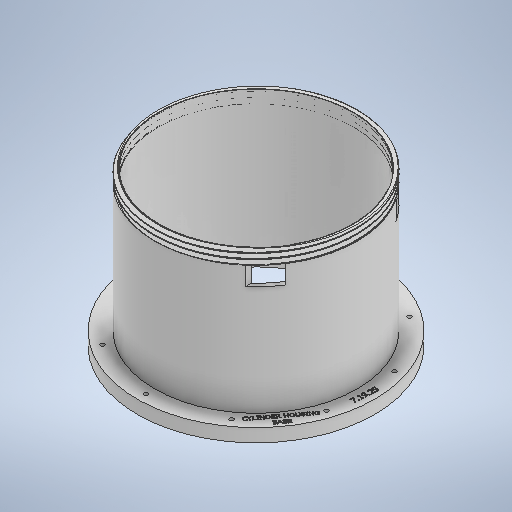
# Autodesk Inventor part: Cylinder Housing_base
Saved by Autodesk Inventor 2025 (Build 290162000, 162)
## iProperties
Created: 2025-07-09
Part Number: Cylinder Housing_base
Material: Generic
Document SubType Name: Modeling
Designer: mumin
Density: 1 g/cm^3
Appearance: Default
Author: mumin
Autodesk Inventor part; units mm, degrees
ref_plane "YZ Plane" through (0, 0, 0) normal (1, 0, 0) x (0, 1, 0)
ref_plane "XZ Plane" through (0, 0, 0) normal (0, 1, 0) x (-1, 0, 0)
ref_plane "XY Plane" through (0, 0, 0) normal (0, 0, 1) x (1, 0, 0)
sketch "Sketch1" plane through (0, 0, 0) normal (0, 0, 1) x (1, 0, 0)
  line L0 (110, 0) -> (110, 175)
  line L1 (110, 0) -> (135, 0)
  line L2 (135, 0) -> (135, 15)
  line L3 (135, 15) -> (115, 15)
  line L4 (115, 15) -> (115, 175)
  line L5 (0, -40) -> (0, 240) projected
  line L6 (-27, 0) -> (162, 0) projected
  line L7 (0, 200) -> (0, 195)
  line L8 (110, 175) -> (115, 175)
  point P0 (0, 0)
  point P1 (115, 132.5)
  point P2 (110, 157.9951)
  point P3 (110, 127.5)
  point P4 (112.5, 175)
  dimension "d0" = 135
  dimension "d1" = 110
  dimension "d2" = 115
  dimension "d3" = 15
  dimension "d24" = 175
  constraints: 14 end point, 6 point on line, 4 perpendicular, 1 collinear, 1 horizontal, 1 midpoint, 1 vertical
  measures "d0" distance between parallel lines of L5 L2
  measures "d1" distance between parallel lines of L5 L0
  measures "d2" distance between parallel lines of L5 L4
  measures "d3" distance of L1.end L2.end
  measures "d24" distance from line of L6 point (112.5, 175)
revolve "Revolution1" add sketch "Sketch1" angle 360 about axis through (0, -10, 0) along (0, 1, 0)
sketch "Sketch3" plane through (0, 15, 0) normal (0, 1, 0) x (1, 0, 0)
  point P0 (0, 0)
  point P1 (0, -125)
  dimension "d11" = 125
  measures "d11" distance of point (0, 0) point (0, -125)
hole "Hole1" at (0, 15, 125) direction (0, -1, 0) diameter 4.5 depth 15
pattern_circular "Circular Pattern1" count 10 over 360 about axis through (0, -10, 0) along (0, 1, 0) of "Hole1"
sketch "Sketch4" plane through (0, 15, 0) normal (0, 1, 0) x (1, 0, 0)
  line L0 (76.2861, -94.0142) -> (115.6188, -42.2704) construction
  line L1 (115.6188, -42.2704) -> (120.4379, -45.9335) construction
  line L2 (120.4379, -45.9335) -> (81.1052, -97.6773) construction
  line L3 (81.1052, -97.6773) -> (76.2861, -94.0142) construction
  line L4 (120.7443, -14.9348) -> (122.6586, 12.509) construction
  line L5 (122.6586, 12.509) -> (135.1331, 11.6389) construction
  line L6 (135.1331, 11.6389) -> (133.2188, -15.805) construction
  line L7 (133.2188, -15.805) -> (120.7443, -14.9348) construction
  spline S0 degree 2 poles (82.4542, -94.4835) (82.16, -94.8706) (81.401, -95.3268) (80.9582, -95.3669) knots 0 0 0 1 2 2 2
  spline S1 degree 2 poles (80.9582, -95.3669) (80.5187, -95.4094) (79.5459, -95.0822) (79.0427, -94.6997) knots 0 0 0 1 2 2 2
  spline S2 degree 2 poles (79.0427, -94.6997) (78.5427, -94.3196) (77.9945, -93.5009) (77.9042, -93.0505) knots 0 0 0 1 2 2 2
  spline S3 degree 2 poles (77.9042, -93.0505) (77.818, -92.6083) (78.0326, -91.7434) (78.3391, -91.3402) knots 0 0 0 1 2 2 2
  spline S4 degree 2 poles (78.3391, -91.3402) (78.4911, -91.1402) (78.8165, -90.8327) (78.9744, -90.7186) knots 0 0 0 1 2 2 2
  spline S5 degree 2 poles (78.9744, -90.7186) (79.1144, -90.6215) (79.4373, -90.4445) (79.6088, -90.3662) knots 0 0 0 1 2 2 2
  line L8 (79.6088, -90.3662) -> (80.2475, -90.8517)
  line L9 (80.2475, -90.8517) -> (80.2156, -90.8936)
  spline S6 degree 2 poles (80.2156, -90.8936) (80.0972, -90.9155) (79.7498, -90.9976) (79.5425, -91.0894) knots 0 0 0 1 2 2 2
  spline S7 degree 2 poles (79.5425, -91.0894) (79.3434, -91.1773) (78.9648, -91.4544) (78.7883, -91.6867) knots 0 0 0 1 2 2 2
  spline S8 degree 2 poles (78.7883, -91.6867) (78.5946, -91.9415) (78.4585, -92.5557) (78.5285, -92.8787) knots 0 0 0 1 2 2 2
  spline S9 degree 2 poles (78.5285, -92.8787) (78.6043, -93.2009) (79.0782, -93.8563) (79.462, -94.1481) knots 0 0 0 1 2 2 2
  spline S10 degree 2 poles (79.462, -94.1481) (79.8717, -94.4595) (80.6116, -94.7115) (80.9447, -94.695) knots 0 0 0 1 2 2 2
  spline S11 degree 2 poles (80.9447, -94.695) (81.269, -94.6768) (81.8098, -94.3805) (82.0011, -94.1289) knots 0 0 0 1 2 2 2
  spline S12 degree 2 poles (82.0011, -94.1289) (82.1752, -93.8998) (82.359, -93.4237) (82.3903, -93.2083) knots 0 0 0 1 2 2 2
  spline S13 degree 2 poles (82.3903, -93.2083) (82.4168, -92.9994) (82.4069, -92.6509) (82.3922, -92.543) knots 0 0 0 1 2 2 2
  line L10 (82.3922, -92.543) -> (82.4216, -92.5043)
  line L11 (82.4216, -92.5043) -> (83.0539, -92.9849)
  spline S14 degree 2 poles (83.0539, -92.9849) (83.0146, -93.1637) (82.951, -93.4818) (82.8775, -93.6856) knots 0 0 0 1 2 2 2
  spline S15 degree 2 poles (82.8775, -93.6856) (82.8032, -93.9039) (82.6357, -94.2448) (82.4542, -94.4835) knots 0 0 0 1 2 2 2
  line L12 (81.838, -86.8845) -> (83.0348, -89.9166)
  line L13 (83.0348, -89.9166) -> (84.796, -91.2554)
  line L14 (84.796, -91.2554) -> (84.3939, -91.7845)
  line L15 (84.3939, -91.7845) -> (82.6875, -90.4873)
  line L16 (82.6875, -90.4873) -> (79.3909, -90.1038)
  line L17 (79.3909, -90.1038) -> (79.8372, -89.5167)
  line L18 (79.8372, -89.5167) -> (82.3709, -89.8192)
  line L19 (82.3709, -89.8192) -> (81.4113, -87.4458)
  line L20 (81.4113, -87.4458) -> (81.838, -86.8845)
  line L21 (87.8512, -87.2362) -> (86.0981, -89.5426)
  line L22 (86.0981, -89.5426) -> (82.1175, -86.5168)
  line L23 (82.1175, -86.5168) -> (82.5196, -85.9878)
  line L24 (82.5196, -85.9878) -> (86.0292, -88.6556)
  line L25 (86.0292, -88.6556) -> (87.3803, -86.8782)
  line L26 (87.3803, -86.8782) -> (87.8512, -87.2362)
  line L27 (89.2219, -85.433) -> (88.0499, -86.9749)
  line L28 (88.0499, -86.9749) -> (87.6434, -86.666)
  line L29 (87.6434, -86.666) -> (88.0284, -86.1595)
  line L30 (88.0284, -86.1595) -> (84.8607, -83.7516)
  line L31 (84.8607, -83.7516) -> (84.4758, -84.2581)
  line L32 (84.4758, -84.2581) -> (84.0693, -83.9491)
  line L33 (84.0693, -83.9491) -> (85.2414, -82.4072)
  line L34 (85.2414, -82.4072) -> (85.6478, -82.7162)
  line L35 (85.6478, -82.7162) -> (85.2629, -83.2226)
  line L36 (85.2629, -83.2226) -> (88.4305, -85.6305)
  line L37 (88.4305, -85.6305) -> (88.8155, -85.1241)
  line L38 (88.8155, -85.1241) -> (89.2219, -85.433)
  line L39 (91.8848, -81.9299) -> (91.4336, -82.5234)
  line L40 (91.4336, -82.5234) -> (86.6627, -81.6757)
  line L41 (86.6627, -81.6757) -> (90.0948, -84.2847)
  line L42 (90.0948, -84.2847) -> (89.7197, -84.7782)
  line L43 (89.7197, -84.7782) -> (85.7391, -81.7524)
  line L44 (85.7391, -81.7524) -> (86.3104, -81.0008)
  line L45 (86.3104, -81.0008) -> (90.6806, -81.7933)
  line L46 (90.6806, -81.7933) -> (87.5291, -79.3976)
  line L47 (87.5291, -79.3976) -> (87.9043, -78.9041)
  line L48 (87.9043, -78.9041) -> (91.8848, -81.9299)
  spline S16 degree 2 poles (92.8966, -76.4744) (93.4417, -76.8888) (93.9832, -77.9977) (93.9463, -78.555) knots 0 0 0 1 2 2 2
  spline S17 degree 2 poles (93.9463, -78.555) (93.9062, -79.0028) (93.562, -79.7235) (93.1942, -80.2073) knots 0 0 0 1 2 2 2
  line L49 (93.1942, -80.2073) -> (92.4978, -81.1235)
  line L50 (92.4978, -81.1235) -> (88.5173, -78.0977)
  line L51 (88.5173, -78.0977) -> (89.2063, -77.1913)
  spline S18 degree 2 poles (89.2063, -77.1913) (89.6329, -76.63) (90.2862, -76.1188) (90.6062, -76.0058) knots 0 0 0 1 2 2 2
  spline S19 degree 2 poles (90.6062, -76.0058) (91.1528, -75.8156) (92.3159, -76.033) (92.8966, -76.4744) knots 0 0 0 1 2 2 2
  spline S20 degree 2 poles (92.4708, -77.0211) (92.0128, -76.6729) (91.1339, -76.4833) (90.722, -76.6435) knots 0 0 0 1 2 2 2
  spline S21 degree 2 poles (90.722, -76.6435) (90.4344, -76.7608) (89.9561, -77.1556) (89.6839, -77.5136) knots 0 0 0 1 2 2 2
  line L52 (89.6839, -77.5136) -> (89.3774, -77.9168)
  line L53 (89.3774, -77.9168) -> (92.4419, -80.2462)
  line L54 (92.4419, -80.2462) -> (92.7484, -79.843)
  spline S22 degree 2 poles (92.7484, -79.843) (93.0156, -79.4914) (93.3073, -78.8734) (93.32, -78.542) knots 0 0 0 1 2 2 2
  spline S23 degree 2 poles (93.32, -78.542) (93.3438, -78.1224) (92.9353, -77.3742) (92.4708, -77.0211) knots 0 0 0 1 2 2 2
  line L55 (95.3201, -77.4106) -> (91.3395, -74.3849)
  line L56 (91.3395, -74.3849) -> (93.2325, -71.8946)
  line L57 (93.2325, -71.8946) -> (93.7034, -72.2526)
  line L58 (93.7034, -72.2526) -> (92.2126, -74.2138)
  line L59 (92.2126, -74.2138) -> (93.3029, -75.0426)
  line L60 (93.3029, -75.0426) -> (94.6932, -73.2136)
  line L61 (94.6932, -73.2136) -> (95.1641, -73.5716)
  line L62 (95.1641, -73.5716) -> (93.7738, -75.4006)
  line L63 (93.7738, -75.4006) -> (95.2512, -76.5236)
  line L64 (95.2512, -76.5236) -> (96.742, -74.5624)
  line L65 (96.742, -74.5624) -> (97.213, -74.9204)
  line L66 (97.213, -74.9204) -> (95.3201, -77.4106)
  line L67 (99.996, -71.2592) -> (99.4737, -71.9463)
  line L68 (99.4737, -71.9463) -> (96.9336, -72.0004)
  line L69 (96.9336, -72.0004) -> (96.4727, -72.6068)
  line L70 (96.4727, -72.6068) -> (98.0565, -73.8107)
  line L71 (98.0565, -73.8107) -> (97.6544, -74.3398)
  line L72 (97.6544, -74.3398) -> (93.6738, -71.314)
  line L73 (93.6738, -71.314) -> (94.4536, -70.2882)
  spline S24 degree 2 poles (94.4536, -70.2882) (94.7135, -69.9463) (95.1383, -69.5414) (95.4332, -69.4347) knots 0 0 0 1 2 2 2
  spline S25 degree 2 poles (95.4332, -69.4347) (95.728, -69.328) (96.3345, -69.4073) (96.6474, -69.6452) knots 0 0 0 1 2 2 2
  spline S26 degree 2 poles (96.6474, -69.6452) (97.0829, -69.9762) (97.3348, -70.87) (97.1874, -71.3586) knots 0 0 0 1 2 2 2
  line L74 (97.1874, -71.3586) -> (99.996, -71.2592)
  spline S27 degree 2 poles (96.27, -70.2286) (96.0958, -70.0962) (95.7349, -70.0153) (95.5498, -70.0781) knots 0 0 0 1 2 2 2
  spline S28 degree 2 poles (95.5498, -70.0781) (95.3897, -70.1346) (95.1004, -70.388) (94.9337, -70.6074) knots 0 0 0 1 2 2 2
  line L75 (94.9337, -70.6074) -> (94.534, -71.1332)
  line L76 (94.534, -71.1332) -> (96.0307, -72.2709)
  line L77 (96.0307, -72.2709) -> (96.3838, -71.8064)
  spline S29 degree 2 poles (96.3838, -71.8064) (96.5579, -71.5774) (96.7544, -71.1516) (96.7242, -70.9301) knots 0 0 0 1 2 2 2
  spline S30 degree 2 poles (96.7242, -70.9301) (96.7028, -70.7306) (96.4765, -70.3856) (96.27, -70.2286) knots 0 0 0 1 2 2 2
  line L78 (103.7329, -66.3432) -> (103.3308, -66.8722)
  line L79 (103.3308, -66.8722) -> (101.3824, -65.3912)
  line L80 (101.3824, -65.3912) -> (99.9897, -67.2234)
  line L81 (99.9897, -67.2234) -> (101.938, -68.7044)
  line L82 (101.938, -68.7044) -> (101.5359, -69.2334)
  line L83 (101.5359, -69.2334) -> (97.5553, -66.2077)
  line L84 (97.5553, -66.2077) -> (97.9575, -65.6787)
  line L85 (97.9575, -65.6787) -> (99.5187, -66.8654)
  line L86 (99.5187, -66.8654) -> (100.9115, -65.0332)
  line L87 (100.9115, -65.0332) -> (99.3502, -63.8464)
  line L88 (99.3502, -63.8464) -> (99.7523, -63.3174)
  line L89 (99.7523, -63.3174) -> (103.7329, -66.3432)
  spline S31 degree 2 poles (102.9608, -60.0407) (103.3969, -60.0159) (104.3624, -60.3528) (104.8591, -60.7304) knots 0 0 0 1 2 2 2
  spline S32 degree 2 poles (104.8591, -60.7304) (105.343, -61.0982) (105.9405, -61.9392) (106.0284, -62.3725) knots 0 0 0 1 2 2 2
  spline S33 degree 2 poles (106.0284, -62.3725) (106.1195, -62.8286) (105.8911, -63.678) (105.5945, -64.0683) knots 0 0 0 1 2 2 2
  spline S34 degree 2 poles (105.5945, -64.0683) (105.288, -64.4715) (104.5234, -64.9082) (104.0766, -64.9402) knots 0 0 0 1 2 2 2
  spline S35 degree 2 poles (104.0766, -64.9402) (103.638, -64.9682) (102.6743, -64.6224) (102.184, -64.2497) knots 0 0 0 1 2 2 2
  spline S36 degree 2 poles (102.184, -64.2497) (101.684, -63.8696) (101.1115, -63.0426) (101.0114, -62.6051) knots 0 0 0 1 2 2 2
  spline S37 degree 2 poles (101.0114, -62.6051) (100.9235, -62.1718) (101.1421, -61.315) (101.4462, -60.915) knots 0 0 0 1 2 2 2
  spline S38 degree 2 poles (101.4462, -60.915) (101.7551, -60.5086) (102.5343, -60.0728) (102.9608, -60.0407) knots 0 0 0 1 2 2 2
  spline S39 degree 2 poles (104.4398, -61.282) (104.0463, -60.9829) (103.3067, -60.6904) (102.989, -60.6932) knots 0 0 0 1 2 2 2
  spline S40 degree 2 poles (102.989, -60.6932) (102.6624, -60.6944) (102.1176, -60.9826) (101.9067, -61.26) knots 0 0 0 1 2 2 2
  spline S41 degree 2 poles (101.9067, -61.26) (101.6885, -61.5471) (101.5599, -62.1313) (101.6477, -62.4577) knots 0 0 0 1 2 2 2
  spline S42 degree 2 poles (101.6477, -62.4577) (101.7308, -62.7702) (102.2162, -63.4038) (102.6033, -63.6981) knots 0 0 0 1 2 2 2
  spline S43 degree 2 poles (102.6033, -63.6981) (103.3871, -64.2939) (104.7196, -64.2685) (105.1389, -63.7169) knots 0 0 0 1 2 2 2
  spline S44 degree 2 poles (105.1389, -63.7169) (105.5581, -63.1653) (105.2237, -61.8779) (104.4398, -61.282) knots 0 0 0 1 2 2 2
  spline S45 degree 2 poles (108.4314, -60.3362) (108.1642, -60.6878) (107.5831, -61.0706) (107.2594, -61.1147) knots 0 0 0 1 2 2 2
  spline S46 degree 2 poles (107.2594, -61.1147) (106.8936, -61.1674) (106.183, -60.897) (105.7572, -60.5733) knots 0 0 0 1 2 2 2
  line L90 (105.7572, -60.5733) -> (103.2734, -58.6853)
  line L91 (103.2734, -58.6853) -> (103.6756, -58.1563)
  line L92 (103.6756, -58.1563) -> (106.1594, -60.0443)
  spline S47 degree 2 poles (106.1594, -60.0443) (106.4368, -60.2552) (106.8649, -60.4687) (107.0925, -60.4839) knots 0 0 0 1 2 2 2
  spline S48 degree 2 poles (107.0925, -60.4839) (107.3347, -60.5001) (107.7788, -60.2574) (107.9798, -59.9929) knots 0 0 0 1 2 2 2
  spline S49 degree 2 poles (107.9798, -59.9929) (108.1686, -59.7445) (108.2984, -59.2324) (108.218, -59.0033) knots 0 0 0 1 2 2 2
  spline S50 degree 2 poles (108.218, -59.0033) (108.1424, -58.7881) (107.8254, -58.4351) (107.5576, -58.2316) knots 0 0 0 1 2 2 2
  line L93 (107.5576, -58.2316) -> (105.0609, -56.3337)
  line L94 (105.0609, -56.3337) -> (105.4631, -55.8047)
  line L95 (105.4631, -55.8047) -> (107.9469, -57.6928)
  spline S51 degree 2 poles (107.9469, -57.6928) (108.363, -58.0091) (108.829, -58.628) (108.8704, -58.9954) knots 0 0 0 1 2 2 2
  spline S52 degree 2 poles (108.8704, -58.9954) (108.9128, -59.3279) (108.711, -59.9684) (108.4314, -60.3362) knots 0 0 0 1 2 2 2
  spline S53 degree 2 poles (110.9343, -57.0168) (110.6057, -57.449) (109.9641, -57.9181) (109.6316, -58.0878) knots 0 0 0 1 2 2 2
  line L96 (109.6316, -58.0878) -> (108.9671, -57.5827)
  line L97 (108.9671, -57.5827) -> (108.9965, -57.544)
  spline S54 degree 2 poles (108.9965, -57.544) (109.4402, -57.469) (110.2139, -57.0137) (110.4468, -56.7073) knots 0 0 0 1 2 2 2
  spline S55 degree 2 poles (110.4468, -56.7073) (110.7803, -56.2686) (110.7566, -55.5431) (110.4566, -55.3151) knots 0 0 0 1 2 2 2
  spline S56 degree 2 poles (110.4566, -55.3151) (110.2179, -55.1336) (109.7421, -55.1435) (109.4742, -55.342) knots 0 0 0 1 2 2 2
  spline S57 degree 2 poles (109.4742, -55.342) (109.2829, -55.4866) (108.979, -55.7391) (108.7468, -55.924) knots 0 0 0 1 2 2 2
  spline S58 degree 2 poles (108.7468, -55.924) (108.535, -56.0888) (108.1229, -56.2895) (107.895, -56.3148) knots 0 0 0 1 2 2 2
  spline S59 degree 2 poles (107.895, -56.3148) (107.6696, -56.3368) (107.2117, -56.2026) (106.9795, -56.026) knots 0 0 0 1 2 2 2
  spline S60 degree 2 poles (106.9795, -56.026) (106.4956, -55.6582) (106.4146, -54.4057) (106.8584, -53.8218) knots 0 0 0 1 2 2 2
  spline S61 degree 2 poles (106.8584, -53.8218) (107.1134, -53.4863) (107.6968, -52.9933) (108.0163, -52.8341) knots 0 0 0 1 2 2 2
  line L98 (108.0163, -52.8341) -> (108.6486, -53.3147)
  line L99 (108.6486, -53.3147) -> (108.6192, -53.3534)
  spline S62 degree 2 poles (108.6192, -53.3534) (108.3003, -53.4113) (107.5911, -53.8087) (107.3434, -54.1345) knots 0 0 0 1 2 2 2
  spline S63 degree 2 poles (107.3434, -54.1345) (107.0639, -54.5022) (107.0633, -55.2194) (107.344, -55.4328) knots 0 0 0 1 2 2 2
  spline S64 degree 2 poles (107.344, -55.4328) (107.5956, -55.624) (108.0991, -55.5843) (108.3581, -55.3842) knots 0 0 0 1 2 2 2
  spline S65 degree 2 poles (108.3581, -55.3842) (108.5307, -55.2508) (109.0171, -54.852) (109.1881, -54.7275) knots 0 0 0 1 2 2 2
  spline S66 degree 2 poles (109.1881, -54.7275) (109.6253, -54.4134) (110.4211, -54.4178) (110.792, -54.6997) knots 0 0 0 1 2 2 2
  spline S67 degree 2 poles (110.792, -54.6997) (111.0275, -54.8787) (111.3344, -55.4123) (111.3625, -55.7034) knots 0 0 0 1 2 2 2
  spline S68 degree 2 poles (111.3625, -55.7034) (111.3921, -56.0262) (111.2114, -56.6522) (110.9343, -57.0168) knots 0 0 0 1 2 2 2
  line L100 (113.3913, -53.6371) -> (112.2193, -55.179)
  line L101 (112.2193, -55.179) -> (111.8128, -54.87)
  line L102 (111.8128, -54.87) -> (112.1978, -54.3636)
  line L103 (112.1978, -54.3636) -> (109.0301, -51.9557)
  line L104 (109.0301, -51.9557) -> (108.6452, -52.4622)
  line L105 (108.6452, -52.4622) -> (108.2387, -52.1532)
  line L106 (108.2387, -52.1532) -> (109.4108, -50.6113)
  line L107 (109.4108, -50.6113) -> (109.8172, -50.9203)
  line L108 (109.8172, -50.9203) -> (109.4323, -51.4267)
  line L109 (109.4323, -51.4267) -> (112.5999, -53.8346)
  line L110 (112.5999, -53.8346) -> (112.9849, -53.3281)
  line L111 (112.9849, -53.3281) -> (113.3913, -53.6371)
  line L112 (116.0542, -50.134) -> (115.603, -50.7275)
  line L113 (115.603, -50.7275) -> (110.8321, -49.8798)
  line L114 (110.8321, -49.8798) -> (114.2642, -52.4887)
  line L115 (114.2642, -52.4887) -> (113.8891, -52.9823)
  line L116 (113.8891, -52.9823) -> (109.9086, -49.9565)
  line L117 (109.9086, -49.9565) -> (110.4799, -49.2049)
  line L118 (110.4799, -49.2049) -> (114.85, -49.9973)
  line L119 (114.85, -49.9973) -> (111.6985, -47.6017)
  line L120 (111.6985, -47.6017) -> (112.0737, -47.1082)
  line L121 (112.0737, -47.1082) -> (116.0542, -50.134)
  spline S69 degree 2 poles (118.0123, -47.7187) (117.6911, -48.1413) (116.901, -48.6451) (116.4484, -48.6981) knots 0 0 0 1 2 2 2
  spline S70 degree 2 poles (116.4484, -48.6981) (115.9927, -48.7486) (115.0085, -48.423) (114.5021, -48.038) knots 0 0 0 1 2 2 2
  spline S71 degree 2 poles (114.5021, -48.038) (114.0214, -47.6726) (113.4661, -46.823) (113.3864, -46.3654) knots 0 0 0 1 2 2 2
  spline S72 degree 2 poles (113.3864, -46.3654) (113.3091, -45.9249) (113.5646, -44.9995) (113.8858, -44.5769) knots 0 0 0 1 2 2 2
  spline S73 degree 2 poles (113.8858, -44.5769) (114.0403, -44.3737) (114.3779, -44.0501) (114.557, -43.9216) knots 0 0 0 1 2 2 2
  spline S74 degree 2 poles (114.557, -43.9216) (114.6987, -43.8155) (115.0908, -43.5944) (115.2184, -43.5336) knots 0 0 0 1 2 2 2
  line L122 (115.2184, -43.5336) -> (115.8571, -44.0191)
  line L123 (115.8571, -44.0191) -> (115.8228, -44.0643)
  spline S75 degree 2 poles (115.8228, -44.0643) (115.6596, -44.0981) (115.3422, -44.1876) (115.1048, -44.3125) knots 0 0 0 1 2 2 2
  spline S76 degree 2 poles (115.1048, -44.3125) (114.9015, -44.4125) (114.4788, -44.7477) (114.2973, -44.9864) knots 0 0 0 1 2 2 2
  spline S77 degree 2 poles (114.2973, -44.9864) (113.8609, -45.5605) (114.1859, -46.9273) (114.9052, -47.4741) knots 0 0 0 1 2 2 2
  spline S78 degree 2 poles (114.9052, -47.4741) (115.3052, -47.7782) (116.0474, -48.0472) (116.3887, -48.0267) knots 0 0 0 1 2 2 2
  spline S79 degree 2 poles (116.3887, -48.0267) (116.7251, -48.0126) (117.3091, -47.6931) (117.5396, -47.3899) knots 0 0 0 1 2 2 2
  spline S80 degree 2 poles (117.5396, -47.3899) (117.7087, -47.1673) (117.9826, -46.6731) (118.0333, -46.4724) knots 0 0 0 1 2 2 2
  line L124 (118.0333, -46.4724) -> (117.0043, -45.6903)
  line L125 (117.0043, -45.6903) -> (116.3031, -46.6128)
  line L126 (116.3031, -46.6128) -> (115.8386, -46.2597)
  line L127 (115.8386, -46.2597) -> (116.9371, -44.8146)
  line L128 (116.9371, -44.8146) -> (118.6757, -46.1362)
  spline S81 degree 2 poles (118.6757, -46.1362) (118.6449, -46.2706) (118.5237, -46.7179) (118.4553, -46.8949) knots 0 0 0 1 2 2 2
  spline S82 degree 2 poles (118.4553, -46.8949) (118.3637, -47.1359) (118.1815, -47.4961) (118.0123, -47.7187) knots 0 0 0 1 2 2 2
  spline S83 degree 2 poles (102.9072, -78.4955) (103.204, -78.7211) (103.4872, -79.2927) (103.4933, -79.5925) knots 0 0 0 1 2 2 2
  spline S84 degree 2 poles (103.4933, -79.5925) (103.4959, -79.9507) (103.2544, -80.5764) (102.9454, -80.9829) knots 0 0 0 1 2 2 2
  line L129 (102.9454, -80.9829) -> (102.0774, -82.1248)
  line L130 (102.0774, -82.1248) -> (98.0969, -79.099)
  line L131 (98.0969, -79.099) -> (98.8987, -78.0442)
  spline S85 degree 2 poles (98.8987, -78.0442) (99.2224, -77.6184) (99.6009, -77.2343) (99.8544, -77.1217) knots 0 0 0 1 2 2 2
  spline S86 degree 2 poles (99.8544, -77.1217) (100.1316, -76.9914) (100.6521, -77.0766) (100.9037, -77.2678) knots 0 0 0 1 2 2 2
  spline S87 degree 2 poles (100.9037, -77.2678) (101.1844, -77.4811) (101.4039, -78.1163) (101.3311, -78.4732) knots 0 0 0 1 2 2 2
  line L132 (101.3311, -78.4732) -> (101.3505, -78.4879)
  spline S88 degree 2 poles (101.3505, -78.4879) (101.717, -78.2066) (102.5266, -78.2062) (102.9072, -78.4955) knots 0 0 0 1 2 2 2
  spline S89 degree 2 poles (102.5105, -79.0643) (102.2847, -78.8927) (101.8963, -78.801) (101.6459, -78.9161) knots 0 0 0 1 2 2 2
  spline S90 degree 2 poles (101.6459, -78.9161) (101.4858, -78.9928) (101.2215, -79.2602) (101.0131, -79.5344) knots 0 0 0 1 2 2 2
  line L133 (101.0131, -79.5344) -> (100.557, -80.1344)
  line L134 (100.557, -80.1344) -> (102.0279, -81.2525)
  line L135 (102.0279, -81.2525) -> (102.3541, -80.8235)
  spline S91 degree 2 poles (102.3541, -80.8235) (102.6189, -80.4751) (102.8584, -80.026) (102.8729, -79.7927) knots 0 0 0 1 2 2 2
  spline S92 degree 2 poles (102.8729, -79.7927) (102.8792, -79.5634) (102.7202, -79.2237) (102.5105, -79.0643) knots 0 0 0 1 2 2 2
  spline S93 degree 2 poles (100.5586, -77.8758) (100.4167, -77.7679) (100.1303, -77.7029) (99.988, -77.7627) knots 0 0 0 1 2 2 2
  spline S94 degree 2 poles (99.988, -77.7627) (99.819, -77.8378) (99.5489, -78.1262) (99.3356, -78.4068) knots 0 0 0 1 2 2 2
  line L136 (99.3356, -78.4068) -> (98.9506, -78.9133)
  line L137 (98.9506, -78.9133) -> (100.1151, -79.7984)
  line L138 (100.1151, -79.7984) -> (100.5712, -79.1985)
  spline S95 degree 2 poles (100.5712, -79.1985) (100.76, -78.9501) (100.8874, -78.6754) (100.9023, -78.4883) knots 0 0 0 1 2 2 2
  spline S96 degree 2 poles (100.9023, -78.4883) (100.9181, -78.3068) (100.7457, -78.018) (100.5586, -77.8758) knots 0 0 0 1 2 2 2
  line L139 (104.2033, -79.3281) -> (101.2428, -74.9604)
  line L140 (101.2428, -74.9604) -> (101.7381, -74.3088)
  line L141 (101.7381, -74.3088) -> (106.7387, -75.9927)
  line L142 (106.7387, -75.9927) -> (106.3145, -76.5507)
  line L143 (106.3145, -76.5507) -> (104.927, -76.0661)
  line L144 (104.927, -76.0661) -> (103.7721, -77.5854)
  line L145 (103.7721, -77.5854) -> (104.6103, -78.7926)
  line L146 (104.6103, -78.7926) -> (104.2033, -79.3281)
  line L147 (104.365, -75.8679) -> (102.0226, -75.0594)
  line L148 (102.0226, -75.0594) -> (103.4308, -77.0969)
  line L149 (103.4308, -77.0969) -> (104.365, -75.8679)
  spline S97 degree 2 poles (107.94, -74.5596) (107.6115, -74.9918) (106.9698, -75.4609) (106.6373, -75.6306) knots 0 0 0 1 2 2 2
  line L150 (106.6373, -75.6306) -> (105.9728, -75.1255)
  line L151 (105.9728, -75.1255) -> (106.0022, -75.0868)
  spline S98 degree 2 poles (106.0022, -75.0868) (106.446, -75.0118) (107.2196, -74.5565) (107.4525, -74.2501) knots 0 0 0 1 2 2 2
  spline S99 degree 2 poles (107.4525, -74.2501) (107.786, -73.8114) (107.7623, -73.0859) (107.4624, -72.8579) knots 0 0 0 1 2 2 2
  spline S100 degree 2 poles (107.4624, -72.8579) (107.2236, -72.6765) (106.7479, -72.6863) (106.48, -72.8848) knots 0 0 0 1 2 2 2
  spline S101 degree 2 poles (106.48, -72.8848) (106.2886, -73.0294) (105.9847, -73.2819) (105.7525, -73.4668) knots 0 0 0 1 2 2 2
  spline S102 degree 2 poles (105.7525, -73.4668) (105.5408, -73.6316) (105.1286, -73.8323) (104.9007, -73.8576) knots 0 0 0 1 2 2 2
  spline S103 degree 2 poles (104.9007, -73.8576) (104.6753, -73.8796) (104.2175, -73.7454) (103.9852, -73.5688) knots 0 0 0 1 2 2 2
  spline S104 degree 2 poles (103.9852, -73.5688) (103.5014, -73.201) (103.4203, -71.9485) (103.8641, -71.3646) knots 0 0 0 1 2 2 2
  spline S105 degree 2 poles (103.8641, -71.3646) (104.1192, -71.0291) (104.7026, -70.5361) (105.0221, -70.3769) knots 0 0 0 1 2 2 2
  line L152 (105.0221, -70.3769) -> (105.6543, -70.8575)
  line L153 (105.6543, -70.8575) -> (105.6249, -70.8962)
  spline S106 degree 2 poles (105.6249, -70.8962) (105.306, -70.9541) (104.5968, -71.3515) (104.3492, -71.6773) knots 0 0 0 1 2 2 2
  spline S107 degree 2 poles (104.3492, -71.6773) (104.0696, -72.045) (104.0691, -72.7622) (104.3497, -72.9756) knots 0 0 0 1 2 2 2
  spline S108 degree 2 poles (104.3497, -72.9756) (104.6013, -73.1668) (105.1048, -73.1271) (105.3638, -72.927) knots 0 0 0 1 2 2 2
  spline S109 degree 2 poles (105.3638, -72.927) (105.5365, -72.7936) (106.0228, -72.3948) (106.1938, -72.2703) knots 0 0 0 1 2 2 2
  spline S110 degree 2 poles (106.1938, -72.2703) (106.631, -71.9562) (107.4268, -71.9606) (107.7978, -72.2426) knots 0 0 0 1 2 2 2
  spline S111 degree 2 poles (107.7978, -72.2426) (108.0333, -72.4216) (108.3402, -72.9551) (108.3683, -73.2463) knots 0 0 0 1 2 2 2
  spline S112 degree 2 poles (108.3683, -73.2463) (108.3978, -73.569) (108.2171, -74.1951) (107.94, -74.5596) knots 0 0 0 1 2 2 2
  line L154 (109.3427, -72.567) -> (105.3622, -69.5412)
  line L155 (105.3622, -69.5412) -> (107.2551, -67.0509)
  line L156 (107.2551, -67.0509) -> (107.7261, -67.4089)
  line L157 (107.7261, -67.4089) -> (106.2353, -69.3702)
  line L158 (106.2353, -69.3702) -> (107.3256, -70.1989)
  line L159 (107.3256, -70.1989) -> (108.7158, -68.37)
  line L160 (108.7158, -68.37) -> (109.1868, -68.728)
  line L161 (109.1868, -68.728) -> (107.7965, -70.5569)
  line L162 (107.7965, -70.5569) -> (109.2739, -71.68)
  line L163 (109.2739, -71.68) -> (110.7647, -69.7187)
  line L164 (110.7647, -69.7187) -> (111.2357, -70.0767)
  line L165 (111.2357, -70.0767) -> (109.3427, -72.567)
  line L166 (122.0604, -10.8106) -> (126.9679, -13.7556)
  line L167 (126.9679, -13.7556) -> (126.9083, -14.6093)
  line L168 (126.9083, -14.6093) -> (121.817, -11.5052)
  line L169 (121.817, -11.5052) -> (121.6015, -14.595)
  line L170 (121.6015, -14.595) -> (120.8982, -14.5459)
  line L171 (120.8982, -14.5459) -> (121.1631, -10.748)
  line L172 (121.1631, -10.748) -> (122.0604, -10.8106)
  line L173 (127.2893, -9.1477) -> (127.2223, -10.1081)
  line L174 (127.2223, -10.1081) -> (126.0776, -10.0282)
  line L175 (126.0776, -10.0282) -> (126.1446, -9.0679)
  line L176 (126.1446, -9.0679) -> (127.2893, -9.1477)
  line L177 (127.61, -4.5495) -> (127.4063, -7.4694)
  line L178 (127.4063, -7.4694) -> (126.7952, -7.4268)
  line L179 (126.7952, -7.4268) -> (126.871, -6.3403)
  line L180 (126.871, -6.3403) -> (122.8596, -6.0605)
  line L181 (122.8596, -6.0605) -> (122.7839, -7.147)
  line L182 (122.7839, -7.147) -> (122.2357, -7.1088)
  spline S113 degree 2 poles (122.2357, -7.1088) (122.2787, -6.4928) (121.9701, -5.8864) (121.4877, -5.8137) knots 0 0 0 1 2 2 2
  line L183 (121.4877, -5.8137) -> (121.5311, -5.1929)
  line L184 (121.5311, -5.1929) -> (126.9248, -5.5691)
  line L185 (126.9248, -5.5691) -> (126.9988, -4.5068)
  line L186 (126.9988, -4.5068) -> (127.61, -4.5495)
  spline S114 degree 2 poles (123.6349, -3.3315) (123.1741, -3.2994) (122.4287, -2.9452) (122.1705, -2.664) knots 0 0 0 1 2 2 2
  spline S115 degree 2 poles (122.1705, -2.664) (121.921, -2.398) (121.6755, -1.6546) (121.7012, -1.286) knots 0 0 0 1 2 2 2
  spline S116 degree 2 poles (121.7012, -1.286) (121.73, -0.8737) (122.0531, -0.2236) (122.3323, 0.0055) knots 0 0 0 1 2 2 2
  spline S117 degree 2 poles (122.3323, 0.0055) (122.6838, 0.2929) (123.7746, 0.558) (124.5943, 0.5008) knots 0 0 0 1 2 2 2
  spline S118 degree 2 poles (124.5943, 0.5008) (125.3364, 0.449) (126.6421, 0.0217) (127.0608, -0.3341) knots 0 0 0 1 2 2 2
  spline S119 degree 2 poles (127.0608, -0.3341) (127.5024, -0.711) (127.9247, -1.7152) (127.8753, -2.4234) knots 0 0 0 1 2 2 2
  spline S120 degree 2 poles (127.8753, -2.4234) (127.8641, -2.5835) (127.8048, -2.9449) (127.7455, -3.0967) knots 0 0 0 1 2 2 2
  line L187 (127.7455, -3.0967) -> (126.9742, -3.0429)
  line L188 (126.9742, -3.0429) -> (126.9769, -3.0041)
  spline S121 degree 2 poles (126.9769, -3.0041) (127.0422, -2.9063) (127.1739, -2.4866) (127.1891, -2.2683) knots 0 0 0 1 2 2 2
  spline S122 degree 2 poles (127.1891, -2.2683) (127.2439, -1.4825) (126.2685, -0.5128) (125.3125, -0.3827) knots 0 0 0 1 2 2 2
  spline S123 degree 2 poles (125.3125, -0.3827) (125.5085, -0.7181) (125.6667, -1.314) (125.6427, -1.6584) knots 0 0 0 1 2 2 2
  spline S124 degree 2 poles (125.6427, -1.6584) (125.6197, -1.9882) (125.436, -2.5262) (125.2081, -2.7881) knots 0 0 0 1 2 2 2
  spline S125 degree 2 poles (125.2081, -2.7881) (124.9384, -3.091) (124.1636, -3.3684) (123.6349, -3.3315) knots 0 0 0 1 2 2 2
  spline S126 degree 2 poles (124.3583, -0.2967) (123.752, -0.2544) (122.9701, -0.4241) (122.7476, -0.6084) knots 0 0 0 1 2 2 2
  spline S127 degree 2 poles (122.7476, -0.6084) (122.5415, -0.7695) (122.3706, -1.1231) (122.3557, -1.3365) knots 0 0 0 1 2 2 2
  spline S128 degree 2 poles (122.3557, -1.3365) (122.3212, -1.8313) (122.9884, -2.4676) (123.6578, -2.5143) knots 0 0 0 1 2 2 2
  spline S129 degree 2 poles (123.6578, -2.5143) (124.0361, -2.5407) (124.5395, -2.3808) (124.729, -2.1796) knots 0 0 0 1 2 2 2
  spline S130 degree 2 poles (124.729, -2.1796) (124.866, -2.0331) (124.9751, -1.6557) (124.9907, -1.4326) knots 0 0 0 1 2 2 2
  spline S131 degree 2 poles (124.9907, -1.4326) (125.0086, -1.1755) (124.8705, -0.5712) (124.7357, -0.3376) knots 0 0 0 1 2 2 2
  spline S132 degree 2 poles (124.7357, -0.3376) (124.6778, -0.3287) (124.4796, -0.3052) (124.3583, -0.2967) knots 0 0 0 1 2 2 2
  line L189 (128.0897, 2.3285) -> (128.0228, 1.3681)
  line L190 (128.0228, 1.3681) -> (126.8781, 1.4479)
  line L191 (126.8781, 1.4479) -> (126.945, 2.4083)
  line L192 (126.945, 2.4083) -> (128.0897, 2.3285)
  line L193 (128.4315, 7.2274) -> (128.174, 3.5362)
  line L194 (128.174, 3.5362) -> (127.3252, 3.5954)
  spline S133 degree 2 poles (127.3252, 3.5954) (126.9794, 4.0192) (126.3352, 4.7758) (125.9854, 5.1414) knots 0 0 0 1 2 2 2
  spline S134 degree 2 poles (125.9854, 5.1414) (125.2813, 5.8777) (124.4139, 6.4402) (123.9338, 6.4737) knots 0 0 0 1 2 2 2
  spline S135 degree 2 poles (123.9338, 6.4737) (123.6815, 6.4913) (123.2924, 6.3625) (123.1613, 6.2303) knots 0 0 0 1 2 2 2
  spline S136 degree 2 poles (123.1613, 6.2303) (123.0302, 6.0981) (122.8832, 5.7379) (122.8677, 5.5148) knots 0 0 0 1 2 2 2
  spline S137 degree 2 poles (122.8677, 5.5148) (122.8528, 5.3014) (122.9291, 4.8574) (122.9976, 4.6528) knots 0 0 0 1 2 2 2
  spline S138 degree 2 poles (122.9976, 4.6528) (123.0537, 4.4783) (123.2257, 4.1495) (123.2869, 4.0477) knots 0 0 0 1 2 2 2
  line L195 (123.2869, 4.0477) -> (123.2838, 4.0041)
  line L196 (123.2838, 4.0041) -> (122.4302, 4.0636)
  spline S139 degree 2 poles (122.4302, 4.0636) (122.3261, 4.3194) (122.1504, 5.2236) (122.1781, 5.6214) knots 0 0 0 1 2 2 2
  spline S140 degree 2 poles (122.1781, 5.6214) (122.2367, 6.4605) (123.1903, 7.3444) (123.9469, 7.2917) knots 0 0 0 1 2 2 2
  spline S141 degree 2 poles (123.9469, 7.2917) (124.301, 7.267) (124.8813, 7.0608) (125.1233, 6.8977) knots 0 0 0 1 2 2 2
  spline S142 degree 2 poles (125.1233, 6.8977) (125.3751, 6.7339) (125.8598, 6.276) (126.091, 6.0259) knots 0 0 0 1 2 2 2
  spline S143 degree 2 poles (126.091, 6.0259) (126.4769, 5.6189) (127.295, 4.6308) (127.5328, 4.3364) knots 0 0 0 1 2 2 2
  line L197 (127.5328, 4.3364) -> (127.7378, 7.2758)
  line L198 (127.7378, 7.2758) -> (128.4315, 7.2274)
  spline S144 degree 2 poles (126.839, 11.7885) (127.2707, 11.7584) (127.9886, 11.4305) (128.2427, 11.1593) knots 0 0 0 1 2 2 2
  spline S145 degree 2 poles (128.2427, 11.1593) (128.4967, 10.8882) (128.7596, 10.1144) (128.7271, 9.6487) knots 0 0 0 1 2 2 2
  spline S146 degree 2 poles (128.7271, 9.6487) (128.6973, 9.2219) (128.4499, 8.4008) (128.2783, 8.1057) knots 0 0 0 1 2 2 2
  line L199 (128.2783, 8.1057) -> (127.4294, 8.1649)
  line L200 (127.4294, 8.1649) -> (127.4335, 8.2231)
  spline S147 degree 2 poles (127.4335, 8.2231) (127.5078, 8.3105) (127.7065, 8.6427) (127.7986, 8.8459) knots 0 0 0 1 2 2 2
  spline S148 degree 2 poles (127.7986, 8.8459) (127.8977, 9.0778) (128.0172, 9.4643) (128.0345, 9.7116) knots 0 0 0 1 2 2 2
  spline S149 degree 2 poles (128.0345, 9.7116) (128.0514, 9.9542) (127.9086, 10.4223) (127.7309, 10.6004) knots 0 0 0 1 2 2 2
  spline S150 degree 2 poles (127.7309, 10.6004) (127.5619, 10.7633) (127.0974, 10.9516) (126.7773, 10.974) knots 0 0 0 1 2 2 2
  spline S151 degree 2 poles (126.7773, 10.974) (126.4572, 10.9963) (126.0375, 10.8501) (125.8902, 10.6947) knots 0 0 0 1 2 2 2
  spline S152 degree 2 poles (125.8902, 10.6947) (125.728, 10.5354) (125.5667, 10.0397) (125.5454, 9.7342) knots 0 0 0 1 2 2 2
  spline S153 degree 2 poles (125.5454, 9.7342) (125.5224, 9.4043) (125.5786, 8.7424) (125.6084, 8.5405) knots 0 0 0 1 2 2 2
  line L201 (125.6084, 8.5405) -> (122.5235, 8.7557)
  line L202 (122.5235, 8.7557) -> (122.7525, 12.0394)
  line L203 (122.7525, 12.0394) -> (123.4558, 11.9904)
  line L204 (123.4558, 11.9904) -> (123.2806, 9.4778)
  line L205 (123.2806, 9.4778) -> (124.8764, 9.3665)
  spline S154 degree 2 poles (124.8764, 9.3665) (124.8671, 9.5134) (124.8722, 9.7957) (124.8803, 9.9121) knots 0 0 0 1 2 2 2
  spline S155 degree 2 poles (124.8803, 9.9121) (124.9125, 10.3729) (125.1072, 10.9979) (125.3506, 11.2733) knots 0 0 0 1 2 2 2
  spline S156 degree 2 poles (125.3506, 11.2733) (125.5943, 11.5536) (126.2957, 11.8264) (126.839, 11.7885) knots 0 0 0 1 2 2 2
  point P0 (0, 0)
  constraints: 4 other
emboss "Emboss1" sketch "Sketch4" operation cut depth 1 direction (0, -1, 0)
thread "Thread1" size "M230x6" class "6g" standard "ANSI Metric M Profile" length 14.5
sketch "Sketch8" plane through (0, 175, 0) normal (1, 0, 0) x (0, 0, 1)
  line L0 (115, 0) -> (115, 14.5)
  line L1 (115, 14.5) -> (110.5512, 14.5)
  line L2 (110.5512, 14.5) -> (110.5512, 0)
  line L3 (110.5512, 0) -> (115, 0)
  line L4 (0, -2.9) -> (0, 17.4) projected
  constraints: 8 end point
revolve "Revolution2" cut sketch "Sketch8" angle 360 about axis through (0, 175, 0) along (0, -1, 0)
sketch "Sketch9" plane through (0, 175, 0) normal (1, 0, 0) x (0, 0, 1)
  line L0 (115, 0) -> (115, 14.5)
  line L1 (115, 14.5) -> (110.5512, 14.5)
  line L2 (110.5512, 14.5) -> (110.5512, 0)
  line L3 (110.5512, 0) -> (115, 0)
  line L4 (0, -2.9) -> (0, 17.4) projected
  constraints: 8 end point
revolve "Revolution3" add sketch "Sketch9" angle 360 about axis through (0, 175, 0) along (0, -1, 0) separate body
sketch "Sketch7" plane through (0, 175, 0) normal (-1, 0, 0) x (0, -1, 0)
  line L0 (-3.5001, -110.8548) -> (-3.0001, -110.8548) construction
  line L1 (0.4999, -114.6968) -> (-0.0001, -115.6573) construction
  line L2 (-6.0001, -115.6573) -> (-6.5001, -114.6968) construction
  line L3 (-2.5001, -110.8548) -> (-3.0001, -109.8943) construction
  line L4 (-3.0001, -109.8943) -> (-3.5001, -110.8548) construction
  line L5 (-6.0001, -115.6573) -> (-5.5001, -114.6968) construction
  line L6 (-2.5001, -110.8548) -> (-0.5001, -114.6968)
  line L7 (-6.5001, -114.6968) -> (-5.5001, -114.6968) construction
  arc A0 (-6.5001, -114.6968) -> (-6.0001, -115.0002) centre (-6.0001, -114.4365) ccw construction
  line L8 (0.4999, -114.6968) -> (-0.5001, -114.6968) construction
  line L9 (-6.0001, -115.6573) -> (-6.0001, -114.6968) construction
  line L10 (-0.0001, -115.6573) -> (-0.0001, -114.6968) construction
  line L11 (-3.0001, -109.8943) -> (-3.0001, -110.5514) construction
  line L12 (-6.0001, -115.0002) -> (-0.0001, -115.0002)
  arc A1 (-6.0001, -115.0002) -> (-5.5001, -114.6968) centre (-6.0001, -114.4365) ccw
  line L13 (-0.5001, -114.6968) -> (-0.0001, -115.6573) construction
  line L14 (-5.5001, -114.6968) -> (-3.5001, -110.8548)
  line L15 (-0.0001, -0.0002) -> (-0.0001, 0.0177)
  line L16 (-0.0001, 0.0177) -> (-0.0001, -0.0002)
  line L17 (-0.0001, -0.0002) -> (0.0334, -0.0002)
  arc A2 (-0.5001, -114.6968) -> (-0.0001, -115.0002) centre (-0.0001, -114.4365) ccw
  arc A3 (-0.0001, -115.0002) -> (0.4999, -114.6968) centre (-0.0001, -114.4365) ccw construction
  arc A4 (-3.0001, -110.5514) -> (-3.5001, -110.8548) centre (-3.0001, -111.1151) ccw
  arc A5 (-2.5001, -110.8548) -> (-3.0001, -110.5514) centre (-3.0001, -111.1151) ccw
  line L18 (-3.0001, -110.5514) -> (-3.0001, -110.8548) construction
  line L19 (-3.0001, -110.8548) -> (-2.5001, -110.8548) construction
  dimension "d38" = 55
  dimension "d39" = 0.9605
  dimension "d40" = 0.9605
  dimension "Sketch7_ThreadOffset" = 0
  dimension "Sketch7_MajorRadius" = 115
  dimension "d43" = 6
  dimension "Sketch7_MinorRadius" = 110.5512
  constraints: 40 end point, 12 point on circle, 10 parallel, 8 tangent, 6 centre point, 6 collinear, 2 midpoint, 2 point on line, 1 horizontal, 1 perpendicular, 3 other
  measures "d38" angle of L6 L14
  measures "d39" distance of L3.end L0.end
  measures "d40" distance of L1.end L10.end
  measures "Sketch7_ThreadOffset" distance between parallel lines of L15 L10
  measures "Sketch7_MajorRadius" distance from line of L12 L15.start
  measures "d43" distance from line of L1.end L9
  measures "Sketch7_MinorRadius" distance edge to line of A5 L17
coil "Coil1" sketch "Sketch7" operation cut axis through (0, 175, 0) along (0, -1, 0) pitch 6.006 turns 4.412254 hand right bodies 2
sketch "Sketch11" plane through (0, 0, 0) normal (0, 0, 1) x (1, 0, 0)
  line L0 (96.16, 139.5) -> (75.16, 139.5)
  line L1 (75.16, 139.5) -> (75.16, 179.5)
  line L2 (75.16, 179.5) -> (96.16, 179.5)
  line L3 (96.16, 179.5) -> (96.16, 139.5)
  line L4 (135, 0) -> (-135, 0) projected
  line L5 (0, -35.9) -> (0, 215.4) projected
  point P0 (0, 0)
  point P1 (85.66, 179.5)
  dimension "d62" = 21
  dimension "d63" = 40
  dimension "d64" = 139.5
  dimension "d65" = 85.66
  constraints: 8 end point, 2 parallel, 1 horizontal, 1 midpoint, 1 perpendicular
  measures "d62" distance of L1.end L2.end
  measures "d63" distance of L0.end L1.end
  measures "d64" distance between parallel lines of L4 L0
  measures "d65" distance from line of L5 point (85.66, 179.5)
extrude "Extrusion4" cut sketch "Sketch11" along normal through all both and the other way through all bodies 1
equation "\"d38\" = d45"
equation "\"d39\" = 0.160083 * Sketch7_Pitch"
equation "\"d40\" = 0.160083 * Sketch7_Pitch"
equation "\"d43\" = Sketch7_Pitch"
equation "\"d45\" = 55deg"
equation "\"Sketch7_Pitch\" = 6"
body "Solid1"
body "Solid2"
